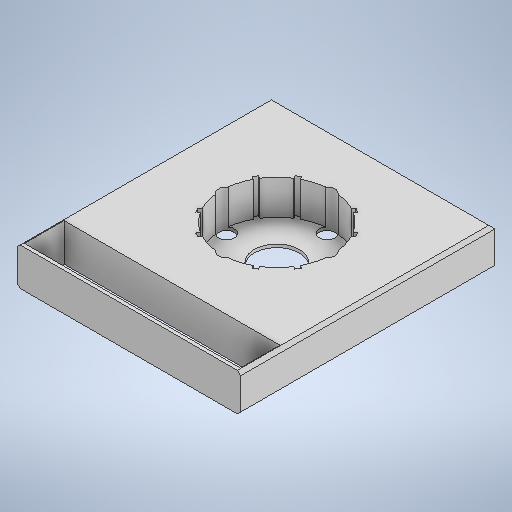
# Autodesk Inventor part: 2024_08_27_Reaktorkorpus_unten
Saved by Autodesk Inventor 2025.1 (Build 291241000, 241)
## iProperties
Created: 2024-08-20
Part Number: 2024_08_27_Reaktorkorpus_unten
Material: Generisch
Document SubType Name: Modeling
Designer: to86hug
Density: 1 g/cm^3
Appearance: Vorgabe
Author: to86hug
Autodesk Inventor part; units mm, degrees
ref_plane "YZ Plane" through (0, 0, 0) normal (1, 0, 0) x (0, 1, 0)
ref_plane "XZ Plane" through (0, 0, 0) normal (0, 1, 0) x (-1, 0, 0)
ref_plane "XY Plane" through (0, 0, 0) normal (0, 0, 1) x (1, 0, 0)
sketch "Skizze1" plane through (0, 0, 0) normal (0, 0, 1) x (1, 0, 0)
  line L0 (70.55, -93.45) -> (70.55, 67.35)
  line L1 (-70.6, -93.45) -> (-70.75, -93.45)
  line L2 (70.55, 67.35) -> (-70.75, 67.35)
  line L3 (-70.75, 67.35) -> (-70.75, -93.45)
  line L4 (-70.75, -93.45) -> (70.55, -93.45)
  line L5 (70.55, -93.45) -> (70.55, 67.35)
  line L6 (-68.25, -66.25) -> (68.25, -66.25)
  line L7 (68.25, -66.25) -> (-68.25, -66.25)
  line L8 (-68.25, -66.25) -> (-68.25, -91.25)
  line L9 (-68.25, -91.25) -> (68.25, -91.25)
  line L10 (68.25, -91.25) -> (68.25, -66.25)
  circle A0 centre (0, 0) radius 14.25
  circle A1 centre (0, 0) radius 14.25
  line L11 (-68.25, -91.25) -> (-68.25, -93.45)
  point P0 (-0.1, -93.25)
  point P1 (70.55, -93.45)
  dimension "d21" = 25
  dimension "d22" = 160.8
  dimension "d23" = 141.3
  dimension "d24" = 28.5
  dimension "d25" = 2.2
  constraints: 24 end point, 4 parallel, 3 perpendicular, 2 centre point, 2 horizontal, 1 coincident, 1 point on line
  measures "d21" distance of L7.end L8.end
  measures "d22" distance of L2.end L1.end
  measures "d23" distance of L1.end L4.end
  measures "d24" diameter of A0
  measures "d25" distance of L8.end L11.end
extrude "Extrusion1" add sketch "Skizze1" along normal blind 23.85
chamfer "Fasen1" distance 2 angle 45 6 edges at (-0.1, 67.35, 23.85) (70.55, -13.05, 23.85) (-70.75, -13.05, 23.85) (70.55, -13.05, 0) (-0.1, 67.35, 0) (-70.75, -13.05, 0)
sketch "Skizze2" plane through (0, 0, 23.85) normal (0, 0, 1) x (1, 0, 0)
  circle A0 centre (0, 0) radius 35.025
  point P0 (0, 1.7417)
  point P1 (0, 1.7417)
  dimension "d5" = 70.05
  constraints: 2 coincident, 1 centre point
  measures "d5" diameter of A0
extrude "Extrusion2" cut sketch "Skizze2" against normal blind 21.9
sketch "Skizze3" plane through (0, 0, 23.85) normal (0, 0, 1) x (1, 0, 0)
  circle A0 centre (31.75, 0) radius 3
  circle A1 centre (31.75, 0) radius 5
  circle A2 centre (0, 0) radius 11.25
  circle A3 centre (0, 0) radius 11.25
  circle A4 centre (0, 31.75) radius 5
  circle A5 centre (-31.75, 0) radius 5
  circle A6 centre (0, -31.75) radius 5
  dimension "d10" = 10
  dimension "d11" = 360
  constraints: 7 centre point, 2 coincident, 9 other
  measures "d10" diameter of A1
extrude "Extrusion3" cut sketch "Skizze3" against normal through all contours A0 | A1 | A4 | A5 | A6
sketch "Skizze4" plane through (0, 0, 23.85) normal (0, 0, 1) x (1, 0, 0)
  line L0 (1.5, -37) -> (-1.5, -37)
  line L1 (-1.5, -37) -> (-1.5, 37)
  line L2 (-1.5, 37) -> (1.5, 37)
  line L3 (1.5, 37) -> (1.5, -37)
  circle A0 centre (0, 0) radius 11.25
  line L4 (1.5, -37) -> (-1.5, 37) construction
  line L5 (-1.5, -37) -> (1.5, 37) construction
  line L6 (0, 0) -> (-1.5, 0)
  line L7 (0, 0) -> (1.5, 0)
  line L8 (17.201, -32.7929) -> (-19.799, 31.2929)
  line L9 (-17.201, 32.7929) -> (19.799, -31.2929)
  line L10 (-19.799, 31.2929) -> (-17.201, 32.7929)
  line L11 (19.799, -31.2929) -> (17.201, -32.7929)
  line L12 (31.2929, -19.799) -> (-32.7929, 17.201)
  line L13 (-31.2929, 19.799) -> (32.7929, -17.201)
  line L14 (-32.7929, 17.201) -> (-31.2929, 19.799)
  line L15 (32.7929, -17.201) -> (31.2929, -19.799)
  line L16 (37, -1.5) -> (-37, -1.5)
  line L17 (-37, 1.5) -> (37, 1.5)
  line L18 (-37, -1.5) -> (-37, 1.5)
  line L19 (37, 1.5) -> (37, -1.5)
  line L20 (32.7929, 17.201) -> (-31.2929, -19.799)
  line L21 (-32.7929, -17.201) -> (31.2929, 19.799)
  line L22 (-31.2929, -19.799) -> (-32.7929, -17.201)
  line L23 (31.2929, 19.799) -> (32.7929, 17.201)
  line L24 (19.799, 31.2929) -> (-17.201, -32.7929)
  line L25 (-19.799, -31.2929) -> (17.201, 32.7929)
  line L26 (-17.201, -32.7929) -> (-19.799, -31.2929)
  line L27 (17.201, 32.7929) -> (19.799, 31.2929)
  line L28 (1.5, 37) -> (1.5, -37)
  line L29 (-1.5, -37) -> (-1.5, 37)
  line L30 (1.5, -37) -> (-1.5, -37)
  line L31 (-1.5, 37) -> (1.5, 37)
  line L32 (-17.201, 32.7929) -> (19.799, -31.2929)
  line L33 (17.201, -32.7929) -> (-19.799, 31.2929)
  line L34 (19.799, -31.2929) -> (17.201, -32.7929)
  line L35 (-19.799, 31.2929) -> (-17.201, 32.7929)
  line L36 (-31.2929, 19.799) -> (32.7929, -17.201)
  line L37 (31.2929, -19.799) -> (-32.7929, 17.201)
  line L38 (32.7929, -17.201) -> (31.2929, -19.799)
  line L39 (-32.7929, 17.201) -> (-31.2929, 19.799)
  line L40 (-37, 1.5) -> (37, 1.5)
  line L41 (37, -1.5) -> (-37, -1.5)
  line L42 (37, 1.5) -> (37, -1.5)
  line L43 (-37, -1.5) -> (-37, 1.5)
  line L44 (-32.7929, -17.201) -> (31.2929, 19.799)
  line L45 (32.7929, 17.201) -> (-31.2929, -19.799)
  line L46 (31.2929, 19.799) -> (32.7929, 17.201)
  line L47 (-31.2929, -19.799) -> (-32.7929, -17.201)
  line L48 (-19.799, -31.2929) -> (17.201, 32.7929)
  line L49 (19.799, 31.2929) -> (-17.201, -32.7929)
  line L50 (17.201, 32.7929) -> (19.799, 31.2929)
  line L51 (-17.201, -32.7929) -> (-19.799, -31.2929)
  circle A1 centre (0, 0) radius 37.0304
  point P0 (0, 0)
  point P1 (-1.299, -0.75)
  point P2 (1.299, 0.75)
  point P3 (-0.75, -1.299)
  point P4 (0.75, 1.299)
  point P5 (0, -1.5)
  point P6 (0, 1.5)
  point P7 (0.75, -1.299)
  point P8 (-0.75, 1.299)
  point P9 (1.299, -0.75)
  point P10 (-1.299, 0.75)
  point P11 (1.5, 0)
  point P12 (-1.5, 0)
  point P13 (1.299, 0.75)
  point P14 (-1.299, -0.75)
  point P15 (0.75, 1.299)
  point P16 (-0.75, -1.299)
  point P17 (0, 1.5)
  point P18 (0, -1.5)
  point P19 (-0.75, 1.299)
  point P20 (0.75, -1.299)
  point P21 (-1.299, 0.75)
  point P22 (1.299, -0.75)
  point P23 (-4.0981, 4.0981)
  point P24 (-3, 0)
  point P25 (-2.049, 0.549)
  point P26 (0, 1.7321)
  point P27 (-0.549, 2.049)
  point P28 (-1.0981, 1.0981)
  point P29 (0.549, 2.049)
  point P30 (1.0981, 1.0981)
  point P31 (31.2929, 19.799)
  point P32 (4.0981, 4.0981)
  point P33 (2.049, 0.549)
  point P34 (3, 0)
  point P35 (-2.049, -0.549)
  point P36 (-4.0981, -4.0981)
  point P37 (-1.0981, -1.0981)
  point P38 (-0.549, -2.049)
  point P39 (0, -1.7321)
  point P40 (2.049, -0.549)
  point P41 (4.0981, -4.0981)
  point P42 (0, 3)
  point P43 (1.7321, 0)
  point P44 (0.549, -2.049)
  point P45 (1.0981, -1.0981)
  point P46 (0, -3)
  point P47 (-1.7321, 0)
  dimension "d16" = 3
  dimension "d17" = 74
  dimension "d18" = 360
  constraints: 104 end point, 4 midpoint, 2 parallel, 1 centre point, 1 coincident, 1 horizontal, 1 perpendicular, 124 other
  measures "d16" distance of L2.start L2.end
  measures "d17" distance of L0.end L2.start
extrude "Extrusion4" cut sketch "Skizze4" against normal up to surface (21.9 mm away) contours L8 A0 L9 L11 | L26 L25 A0 L24 | L8 L24 L12 L3 | L3 L12 L9 A0 L8 | L24 A0 L25 L20 L1 | L1 L20 L8 L24 | L12 A0 L13 L15 | L22 L21 A0 L20 | L9 L16 L13 A0 L12 | L12 L20 L16 L24 | L8 L16 L12 L20 | L20 A0 L21 L16 L25 | L20 L24 L3 | L3 L24 L9 L20 | L9 L20 L13 L16 | L16 L20 L24 | L8 L12 L16 | L12 L25 L8 L1 | L1 L8 L12 | L16 L21 L12 L25 | L9 L3 L13 L24 | L13 L24 L17 L20 | L20 A0 L21 L23 | L8 L21 L1 L25 | L12 L17 L8 L21 | L14 L13 A0 L12 | L9 L13 L3 | L17 L24 L21 A0 L20 | L1 L21 L25 | L12 A0 L13 L8 L17 | L13 L17 L9 | L24 A0 L25 L27 | L25 L17 L21 | L10 L9 A0 L8 | L17 L13 L21 L9 | L21 L3 L25 A0 L24 | L17 L25 L13 L21 | L8 A0 L9 L1 L13 | L21 L9 L25 L3 | L1 L9 L25 L13
